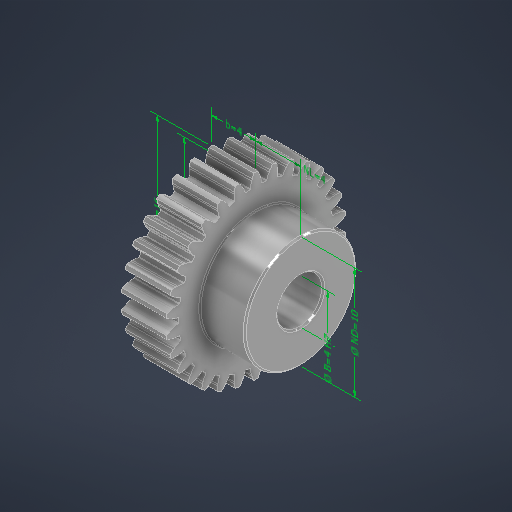
# Autodesk Inventor part: 21103000
Saved by Autodesk Inventor 2026.1 (Build 301233020, 233B)
## iProperties
Category: PARTsolutions
Company: MAEDLER
Created: 2025-12-15
Part Number: 21103000
Material: Generic
Catalog Web Link: www.3dfindit.com
Description: MAE-STZR-M0.5-MN-B4-ST-Spur Gears Made from Steel, with One-Sided Hub, Module 0.5, Tooth Width 4 mm
Vendor: MAEDLER
Document SubType Name: Modeling
Designer: psAdmin
Manufacturer: MAEDLER
Mass: 7 g
Surface Area: 9.18224 cm^2
Volume: 0.913703 cm^3
Density: 1 g/cm^3
Appearance: PSOLRGB-176-176-176
PSOL_IDENT_0: {$CADENAS_DATA/23d-libs/maedler/antriebselemente/stirnzahnraeder/stirnzahnraeder_stahl/modul_0_5_und
PSOL_IDENT_1: _0_7/stzr_m_0_5_zb4_st_mn.prj},173 {VTYP=3D},{NB=21103000},{LINA=21103000},{NN=MAE-STZR-M0.5-MN-B4-S
PSOL_IDENT_2: T},{DATE=31.10.2024 07:34:43},{GEOMDATE=31.10.2024 07:34:43},{VERSION=},{LINEID=190},{WBVAR=},{WBNUM
PSOL_IDENT_3: ERIC=}  {NB=21103000},{LINA=21103000},{KT=DUMMY},{ARTNR=21103000},{WEBSHOP=Produktdetails / Katalogs
PSOL_IDENT_4: eite / Montageanleitung},{MATK=Stahl},{MAT=Stahl 11SMn30+C (1.0715)},{M=0.5},{Z=30},{B=4},{DA=16.0},
PSOL_IDENT_5: {D=15.0},{NL=4},{ND=10},{BH7=4},{MD=5.5},{GEW=7.0},{CTN=84839089},{DIST=0.800},{GKD=14.09539},{FKD=1
PSOL_IDENT_6: 3.83300},{T0=1.57080},{UF=47.12389},{TLG=1.57080},{A=2.56515},{A3=0.85505},{PI=0.39270},{R2=0.04},{C
PSOL_IDENT_7: NSDWTEMPLATE=_dw/ansicht_right_front.dw}
NB: 21103000
NN: MAE-STZR-M0.5-MN-B4-ST
NT: Spur Gears Made from Steel, with One-Sided Hub, Module 0.5, Tooth Width 4 mm
NBSYN: $ARTNR.
LINA: 21103000
CATALOG: MÄDLER
ARTNR: 21103000
WEBSHOP: Product details / Catalogue page / Assembly instructions
MATK: Steel
MAT: Steel 11SMn30+C (1.0715)
M: 0.5
Z: 30
B: 4
DA: 16
D: 15
NL: 4
ND: 10
BH7: 4
MD: 5.5
GEW: 7
CTN: 84839089
SUPPLIER: MAEDLER
ARTICLENO: 21103000
BOMINFO: 21103000
CREATOR: CADENAS GmbH
Title: 21103000
Author: Cadenas PARTsolutions
Comments: Spur Gears Made from Steel, with One-Sided Hub, Module 0.5, Tooth Width 4 mm
Autodesk Inventor part; units mm, degrees
ref_plane "YZ Plane" through (0, 0, 0) normal (1, 0, 0) x (0, 1, 0)
ref_plane "XZ Plane" through (0, 0, 0) normal (0, 1, 0) x (-1, 0, 0)
ref_plane "XY Plane" through (0, 0, 0) normal (0, 0, 1) x (1, 0, 0)
sketch "Sketch_2" plane through (0, 0, 0) normal (0, 0, 1) x (1, 0, 0)
  line L0 (6, 0) -> (-2, 0)
  line L1 (-2, 8) -> (-2, 2.1414)
  line L2 (-2, 2.1414) -> (-1.8586, 2)
  line L3 (-1.8586, 2) -> (5.8586, 2)
  line L4 (5.8586, 2) -> (6, 2.1414)
  line L5 (6, 2.1414) -> (6, 4.8586)
  line L6 (6, 4.8586) -> (5.8586, 5)
  line L7 (5.8586, 5) -> (2.1, 5)
  arc A0 (2, 5.1) -> (2.1, 5) centre (2.1, 5.1) ccw
  line L8 (2, 5.1) -> (2, 8)
  line L9 (2, 8) -> (-2, 8)
  constraints: 20 end point, 2 point on circle, 1 centre point
revolve "Revolution1" add sketch "Sketch_2" angle 360 about axis through (6, 0, 0) along (1, 0, 0)
sketch "Sketch_4" plane through (0, 0, 0) normal (1, 0, 0) x (0, 0, -1)
  circle A0 centre (0, 0) radius 16
  arc A1 (-7.9731, -0.6556) -> (-7.9352, -1.0165) centre (0, 0) ccw
  arc A2 (-7.9352, -1.0165) -> (-7.5578, -1.1394) centre (-6.8326, 1.728) ccw
  arc A3 (-7.5578, -1.1394) -> (-7.4077, -1.1733) centre (-6.9182, 1.3448) ccw
  arc A4 (-7.4077, -1.1733) -> (-6.8456, -1.211) centre (-6.9824, 0.9573) ccw
  arc A5 (-6.8038, -1.2437) -> (-6.8456, -1.211) centre (-6.8431, -1.2509) ccw
  arc A6 (-6.8038, -1.2437) -> (-6.7214, -1.6312) centre (0, 0) ccw
  arc A7 (-6.7463, -1.6781) -> (-6.7214, -1.6312) centre (-6.7603, -1.6406) ccw
  arc A8 (-6.7463, -1.6781) -> (-7.2444, -1.9411) centre (-5.9893, -3.7146) ccw
  arc A9 (-7.2444, -1.9411) -> (-7.3678, -2.0331) centre (-5.7731, -4.0424) ccw
  arc A10 (-7.3678, -2.0331) -> (-7.6626, -2.2989) centre (-5.539, -4.3577) ccw
  arc A11 (-7.6626, -2.2989) -> (-7.5504, -2.6441) centre (0, 0) ccw
  arc A12 (-7.5504, -2.6441) -> (-7.1557, -2.6858) centre (-7.0425, 0.2697) ccw
  arc A13 (-7.1557, -2.6858) -> (-7.0019, -2.6878) centre (-7.0466, -0.123) ccw
  arc A14 (-7.0019, -2.6878) -> (-6.4443, -2.6078) centre (-7.0288, -0.5153) ccw
  arc A15 (-6.3965, -2.6311) -> (-6.4443, -2.6078) centre (-6.4335, -2.6463) ccw
  arc A16 (-6.3965, -2.6311) -> (-6.2354, -2.993) centre (0, 0) ccw
  arc A17 (-6.25, -3.0441) -> (-6.2354, -2.993) centre (-6.2715, -3.0103) ccw
  arc A18 (-6.25, -3.0441) -> (-6.6825, -3.4049) centre (-5.0861, -4.8786) ccw
  arc A19 (-6.6825, -3.4049) -> (-6.7841, -3.5206) centre (-4.8065, -5.1544) ccw
  arc A20 (-6.7841, -3.5206) -> (-7.0171, -3.8418) centre (-4.512, -5.4141) ccw
  arc A21 (-7.0171, -3.8418) -> (-6.8357, -4.1561) centre (0, 0) ccw
  arc A22 (-6.8357, -4.1561) -> (-6.4409, -4.1149) centre (-6.9447, -1.2004) ccw
  arc A23 (-6.4409, -4.1149) -> (-6.29, -4.0848) centre (-6.8671, -1.5854) ccw
  arc A24 (-6.29, -4.0848) -> (-5.7612, -3.8907) centre (-6.7681, -1.9654) ccw
  arc A25 (-5.7097, -3.9035) -> (-5.7612, -3.8907) centre (-5.7427, -3.9261) ccw
  arc A26 (-5.7097, -3.9035) -> (-5.4769, -4.224) centre (0, 0) ccw
  arc A27 (-5.4806, -4.277) -> (-5.4769, -4.224) centre (-5.5085, -4.2484) ccw
  arc A28 (-5.4806, -4.277) -> (-5.8286, -4.7199) centre (-3.9607, -5.8295) ccw
  arc A29 (-5.8286, -4.7199) -> (-5.9039, -4.8541) centre (-3.6298, -6.0411) ccw
  arc A30 (-5.9039, -4.8541) -> (-6.065, -5.2168) centre (-3.2877, -6.2339) ccw
  arc A31 (-6.065, -5.2168) -> (-5.8222, -5.4865) centre (0, 0) ccw
  arc A32 (-5.8222, -5.4865) -> (-5.4446, -5.3641) centre (-6.5434, -2.6181) ccw
  arc A33 (-5.4446, -5.3641) -> (-5.3033, -5.3033) centre (-6.3874, -2.9785) ccw
  arc A34 (-5.3033, -5.3033) -> (-4.8264, -5.0035) centre (-6.2116, -3.3296) ccw
  arc A35 (-4.7733, -5.0053) -> (-4.8264, -5.0035) centre (-4.8009, -5.0343) ccw
  arc A36 (-4.7733, -5.0053) -> (-4.479, -5.2704) centre (0, 0) ccw
  arc A37 (-4.4716, -5.323) -> (-4.479, -5.2704) centre (-4.5049, -5.3009) ccw
  arc A38 (-4.4716, -5.323) -> (-4.7199, -5.8286) centre (-2.6621, -6.5256) ccw
  arc A39 (-4.7199, -5.8286) -> (-4.7656, -5.9755) centre (-2.2945, -6.6637) ccw
  arc A40 (-4.7656, -5.9755) -> (-4.8479, -6.3638) centre (-1.9198, -6.7812) ccw
  arc A41 (-4.8479, -6.3638) -> (-4.5543, -6.5771) centre (0, 0) ccw
  arc A42 (-4.5543, -6.5771) -> (-4.2104, -6.3789) centre (-5.856, -3.9213) ccw
  arc A43 (-4.2104, -6.3789) -> (-4.0848, -6.29) centre (-5.6285, -4.2414) ccw
  arc A44 (-4.0848, -6.29) -> (-3.6807, -5.8976) centre (-5.3836, -4.5483) ccw
  arc A45 (-3.6283, -5.8884) -> (-3.6807, -5.8976) centre (-3.6493, -5.9224) ccw
  arc A46 (-3.6283, -5.8884) -> (-3.2853, -6.0864) centre (0, 0) ccw
  arc A47 (-3.2671, -6.1364) -> (-3.2853, -6.0864) centre (-3.3043, -6.1216) ccw
  arc A48 (-3.2671, -6.1364) -> (-3.4049, -6.6825) centre (-1.2472, -6.9365) ccw
  arc A49 (-3.4049, -6.6825) -> (-3.4191, -6.8358) centre (-0.8589, -6.9952) ccw
  arc A50 (-3.4191, -6.8358) -> (-3.4188, -7.2327) centre (-0.4679, -7.0321) ccw
  arc A51 (-3.4188, -7.2327) -> (-3.0873, -7.3803) centre (0, 0) ccw
  arc A52 (-3.0873, -7.3803) -> (-2.7921, -7.1149) centre (-4.9128, -5.0532) ccw
  arc A53 (-2.7921, -7.1149) -> (-2.6878, -7.0019) centre (-4.6237, -5.319) ccw
  arc A54 (-2.6878, -7.0019) -> (-2.3741, -6.534) centre (-4.3203, -5.5682) ccw
  arc A55 (-2.3248, -6.5141) -> (-2.3741, -6.534) centre (-2.3382, -6.5518) ccw
  arc A56 (-2.3248, -6.5141) -> (-1.9481, -6.6365) centre (0, 0) ccw
  arc A57 (-1.9199, -6.6815) -> (-1.9481, -6.6365) centre (-1.9594, -6.6749) ccw
  arc A58 (-1.9199, -6.6815) -> (-1.9411, -7.2444) centre (0.2222, -7.0442) ccw
  arc A59 (-1.9411, -7.2444) -> (-1.9231, -7.3973) centre (0.6142, -7.0209) ccw
  arc A60 (-1.9231, -7.3973) -> (-1.8403, -7.7854) centre (1.0043, -6.9758) ccw
  arc A61 (-1.8403, -7.7854) -> (-1.4854, -7.8609) centre (0, 0) ccw
  arc A62 (-1.4854, -7.8609) -> (-1.2519, -7.5399) centre (-3.7548, -5.9642) ccw
  arc A63 (-1.2519, -7.5399) -> (-1.1733, -7.4077) centre (-3.4168, -6.1641) ccw
  arc A64 (-1.1733, -7.4077) -> (-0.9637, -6.8848) centre (-3.0682, -6.3448) ccw
  arc A65 (-0.9196, -6.8551) -> (-0.9637, -6.8848) centre (-0.925, -6.8947) ccw
  arc A66 (-0.9196, -6.8551) -> (-0.5257, -6.8965) centre (0, 0) ccw
  arc A67 (-0.4888, -6.9347) -> (-0.5257, -6.8965) centre (-0.5288, -6.9364) ccw
  arc A68 (-0.4888, -6.9347) -> (-0.3925, -7.4897) centre (1.682, -6.8441) ccw
  arc A69 (-0.3925, -7.4897) -> (-0.3431, -7.6355) centre (2.0605, -6.7397) ccw
  arc A70 (-0.3431, -7.6355) -> (-0.1814, -7.9979) centre (2.4327, -6.6145) ccw
  arc A71 (-0.1814, -7.9979) -> (0.1814, -7.9979) centre (0, 0) ccw
  arc A72 (0.1814, -7.9979) -> (0.3431, -7.6355) centre (-2.4327, -6.6145) ccw
  arc A73 (0.3431, -7.6355) -> (0.3925, -7.4897) centre (-2.0605, -6.7397) ccw
  arc A74 (0.3925, -7.4897) -> (0.4888, -6.9347) centre (-1.682, -6.8441) ccw
  arc A75 (0.5257, -6.8965) -> (0.4888, -6.9347) centre (0.5288, -6.9364) ccw
  arc A76 (0.5257, -6.8965) -> (0.9196, -6.8551) centre (0, 0) ccw
  arc A77 (0.9637, -6.8848) -> (0.9196, -6.8551) centre (0.925, -6.8947) ccw
  arc A78 (0.9637, -6.8848) -> (1.1733, -7.4077) centre (3.0682, -6.3448) ccw
  arc A79 (1.1733, -7.4077) -> (1.2519, -7.5399) centre (3.4168, -6.1641) ccw
  arc A80 (1.2519, -7.5399) -> (1.4854, -7.8609) centre (3.7548, -5.9642) ccw
  arc A81 (1.4854, -7.8609) -> (1.8403, -7.7854) centre (0, 0) ccw
  arc A82 (1.8403, -7.7854) -> (1.9231, -7.3973) centre (-1.0043, -6.9758) ccw
  arc A83 (1.9231, -7.3973) -> (1.9411, -7.2444) centre (-0.6142, -7.0209) ccw
  arc A84 (1.9411, -7.2444) -> (1.9199, -6.6815) centre (-0.2222, -7.0442) ccw
  arc A85 (1.9481, -6.6365) -> (1.9199, -6.6815) centre (1.9594, -6.6749) ccw
  arc A86 (1.9481, -6.6365) -> (2.3248, -6.5141) centre (0, 0) ccw
  arc A87 (2.3741, -6.534) -> (2.3248, -6.5141) centre (2.3382, -6.5518) ccw
  arc A88 (2.3741, -6.534) -> (2.6878, -7.0019) centre (4.3203, -5.5682) ccw
  arc A89 (2.6878, -7.0019) -> (2.7921, -7.1149) centre (4.6237, -5.319) ccw
  arc A90 (2.7921, -7.1149) -> (3.0873, -7.3803) centre (4.9128, -5.0532) ccw
  arc A91 (3.0873, -7.3803) -> (3.4188, -7.2327) centre (0, 0) ccw
  arc A92 (3.4188, -7.2327) -> (3.4191, -6.8358) centre (0.4679, -7.0321) ccw
  arc A93 (3.4191, -6.8358) -> (3.4049, -6.6825) centre (0.8589, -6.9952) ccw
  arc A94 (3.4049, -6.6825) -> (3.2671, -6.1364) centre (1.2472, -6.9365) ccw
  arc A95 (3.2853, -6.0864) -> (3.2671, -6.1364) centre (3.3043, -6.1216) ccw
  arc A96 (3.2853, -6.0864) -> (3.6283, -5.8884) centre (0, 0) ccw
  arc A97 (3.6807, -5.8976) -> (3.6283, -5.8884) centre (3.6493, -5.9224) ccw
  arc A98 (3.6807, -5.8976) -> (4.0848, -6.29) centre (5.3836, -4.5483) ccw
  arc A99 (4.0848, -6.29) -> (4.2104, -6.3789) centre (5.6285, -4.2414) ccw
  arc A100 (4.2104, -6.3789) -> (4.5543, -6.5771) centre (5.856, -3.9213) ccw
  arc A101 (4.5543, -6.5771) -> (4.8479, -6.3638) centre (0, 0) ccw
  arc A102 (4.8479, -6.3638) -> (4.7656, -5.9755) centre (1.9198, -6.7812) ccw
  arc A103 (4.7656, -5.9755) -> (4.7199, -5.8286) centre (2.2945, -6.6637) ccw
  arc A104 (4.7199, -5.8286) -> (4.4716, -5.323) centre (2.6621, -6.5256) ccw
  arc A105 (4.479, -5.2704) -> (4.4716, -5.323) centre (4.5049, -5.3009) ccw
  arc A106 (4.479, -5.2704) -> (4.7733, -5.0053) centre (0, 0) ccw
  arc A107 (4.8264, -5.0035) -> (4.7733, -5.0053) centre (4.8009, -5.0343) ccw
  arc A108 (4.8264, -5.0035) -> (5.3033, -5.3033) centre (6.2116, -3.3296) ccw
  arc A109 (5.3033, -5.3033) -> (5.4446, -5.3641) centre (6.3874, -2.9785) ccw
  arc A110 (5.4446, -5.3641) -> (5.8222, -5.4865) centre (6.5434, -2.6181) ccw
  arc A111 (5.8222, -5.4865) -> (6.065, -5.2168) centre (0, 0) ccw
  arc A112 (6.065, -5.2168) -> (5.9039, -4.8541) centre (3.2877, -6.2339) ccw
  arc A113 (5.9039, -4.8541) -> (5.8286, -4.7199) centre (3.6298, -6.0411) ccw
  arc A114 (5.8286, -4.7199) -> (5.4806, -4.277) centre (3.9607, -5.8295) ccw
  arc A115 (5.4769, -4.224) -> (5.4806, -4.277) centre (5.5085, -4.2484) ccw
  arc A116 (5.4769, -4.224) -> (5.7097, -3.9035) centre (0, 0) ccw
  arc A117 (5.7612, -3.8907) -> (5.7097, -3.9035) centre (5.7427, -3.9261) ccw
  arc A118 (5.7612, -3.8907) -> (6.29, -4.0848) centre (6.7681, -1.9654) ccw
  arc A119 (6.29, -4.0848) -> (6.4409, -4.1149) centre (6.8671, -1.5854) ccw
  arc A120 (6.4409, -4.1149) -> (6.8357, -4.1561) centre (6.9447, -1.2004) ccw
  arc A121 (6.8357, -4.1561) -> (7.0171, -3.8418) centre (0, 0) ccw
  arc A122 (7.0171, -3.8418) -> (6.7841, -3.5206) centre (4.512, -5.4141) ccw
  arc A123 (6.7841, -3.5206) -> (6.6825, -3.4049) centre (4.8065, -5.1544) ccw
  arc A124 (6.6825, -3.4049) -> (6.25, -3.0441) centre (5.0861, -4.8786) ccw
  arc A125 (6.2354, -2.993) -> (6.25, -3.0441) centre (6.2715, -3.0103) ccw
  arc A126 (6.2354, -2.993) -> (6.3965, -2.6311) centre (0, 0) ccw
  arc A127 (6.4443, -2.6078) -> (6.3965, -2.6311) centre (6.4335, -2.6463) ccw
  arc A128 (6.4443, -2.6078) -> (7.0019, -2.6878) centre (7.0288, -0.5153) ccw
  arc A129 (7.0019, -2.6878) -> (7.1557, -2.6858) centre (7.0466, -0.123) ccw
  arc A130 (7.1557, -2.6858) -> (7.5504, -2.6441) centre (7.0425, 0.2697) ccw
  arc A131 (7.5504, -2.6441) -> (7.6626, -2.2989) centre (0, 0) ccw
  arc A132 (7.6626, -2.2989) -> (7.3678, -2.0331) centre (5.539, -4.3577) ccw
  arc A133 (7.3678, -2.0331) -> (7.2444, -1.9411) centre (5.7731, -4.0424) ccw
  arc A134 (7.2444, -1.9411) -> (6.7463, -1.6781) centre (5.9893, -3.7146) ccw
  arc A135 (6.7214, -1.6312) -> (6.7463, -1.6781) centre (6.7603, -1.6406) ccw
  arc A136 (6.7214, -1.6312) -> (6.8038, -1.2437) centre (0, 0) ccw
  arc A137 (6.8456, -1.211) -> (6.8038, -1.2437) centre (6.8431, -1.2509) ccw
  arc A138 (6.8456, -1.211) -> (7.4077, -1.1733) centre (6.9824, 0.9573) ccw
  arc A139 (7.4077, -1.1733) -> (7.5578, -1.1394) centre (6.9182, 1.3448) ccw
  arc A140 (7.5578, -1.1394) -> (7.9352, -1.0165) centre (6.8326, 1.728) ccw
  arc A141 (7.9352, -1.0165) -> (7.9731, -0.6556) centre (0, 0) ccw
  arc A142 (7.9731, -0.6556) -> (7.6295, -0.4569) centre (6.324, -3.1108) ccw
  arc A143 (7.6295, -0.4569) -> (7.4897, -0.3925) centre (6.4874, -2.7538) ccw
  arc A144 (7.4897, -0.3925) -> (6.9478, -0.2388) centre (6.6307, -2.3881) ccw
  arc A145 (6.9137, -0.198) -> (6.9478, -0.2388) centre (6.9536, -0.1992) ccw
  arc A146 (6.9137, -0.198) -> (6.9137, 0.198) centre (0, 0) ccw
  arc A147 (6.9478, 0.2388) -> (6.9137, 0.198) centre (6.9536, 0.1992) ccw
  arc A148 (6.9478, 0.2388) -> (7.4897, 0.3925) centre (6.6307, 2.3881) ccw
  arc A149 (7.4897, 0.3925) -> (7.6295, 0.4569) centre (6.4874, 2.7538) ccw
  arc A150 (7.6295, 0.4569) -> (7.9731, 0.6556) centre (6.324, 3.1108) ccw
  arc A151 (7.9731, 0.6556) -> (7.9352, 1.0165) centre (0, 0) ccw
  arc A152 (7.9352, 1.0165) -> (7.5578, 1.1394) centre (6.8326, -1.728) ccw
  arc A153 (7.5578, 1.1394) -> (7.4077, 1.1733) centre (6.9182, -1.3448) ccw
  arc A154 (7.4077, 1.1733) -> (6.8456, 1.211) centre (6.9824, -0.9573) ccw
  arc A155 (6.8038, 1.2437) -> (6.8456, 1.211) centre (6.8431, 1.2509) ccw
  arc A156 (6.8038, 1.2437) -> (6.7214, 1.6312) centre (0, 0) ccw
  arc A157 (6.7463, 1.6781) -> (6.7214, 1.6312) centre (6.7603, 1.6406) ccw
  arc A158 (6.7463, 1.6781) -> (7.2444, 1.9411) centre (5.9893, 3.7146) ccw
  arc A159 (7.2444, 1.9411) -> (7.3678, 2.0331) centre (5.7731, 4.0424) ccw
  arc A160 (7.3678, 2.0331) -> (7.6626, 2.2989) centre (5.539, 4.3577) ccw
  arc A161 (7.6626, 2.2989) -> (7.5504, 2.6441) centre (0, 0) ccw
  arc A162 (7.5504, 2.6441) -> (7.1557, 2.6858) centre (7.0425, -0.2697) ccw
  arc A163 (7.1557, 2.6858) -> (7.0019, 2.6878) centre (7.0466, 0.123) ccw
  arc A164 (7.0019, 2.6878) -> (6.4443, 2.6078) centre (7.0288, 0.5153) ccw
  arc A165 (6.3965, 2.6311) -> (6.4443, 2.6078) centre (6.4335, 2.6463) ccw
  arc A166 (6.3965, 2.6311) -> (6.2354, 2.993) centre (0, 0) ccw
  arc A167 (6.25, 3.0441) -> (6.2354, 2.993) centre (6.2715, 3.0103) ccw
  arc A168 (6.25, 3.0441) -> (6.6825, 3.4049) centre (5.0861, 4.8786) ccw
  arc A169 (6.6825, 3.4049) -> (6.7841, 3.5206) centre (4.8065, 5.1544) ccw
  arc A170 (6.7841, 3.5206) -> (7.0171, 3.8418) centre (4.512, 5.4141) ccw
  arc A171 (7.0171, 3.8418) -> (6.8357, 4.1561) centre (0, 0) ccw
  arc A172 (6.8357, 4.1561) -> (6.4409, 4.1149) centre (6.9447, 1.2004) ccw
  arc A173 (6.4409, 4.1149) -> (6.29, 4.0848) centre (6.8671, 1.5854) ccw
  arc A174 (6.29, 4.0848) -> (5.7612, 3.8907) centre (6.7681, 1.9654) ccw
  arc A175 (5.7097, 3.9035) -> (5.7612, 3.8907) centre (5.7427, 3.9261) ccw
  arc A176 (5.7097, 3.9035) -> (5.4769, 4.224) centre (0, 0) ccw
  arc A177 (5.4806, 4.277) -> (5.4769, 4.224) centre (5.5085, 4.2484) ccw
  arc A178 (5.4806, 4.277) -> (5.8286, 4.7199) centre (3.9607, 5.8295) ccw
  arc A179 (5.8286, 4.7199) -> (5.9039, 4.8541) centre (3.6298, 6.0411) ccw
  arc A180 (5.9039, 4.8541) -> (6.065, 5.2168) centre (3.2877, 6.2339) ccw
  arc A181 (6.065, 5.2168) -> (5.8222, 5.4865) centre (0, 0) ccw
  arc A182 (5.8222, 5.4865) -> (5.4446, 5.3641) centre (6.5434, 2.6181) ccw
  arc A183 (5.4446, 5.3641) -> (5.3033, 5.3033) centre (6.3874, 2.9785) ccw
  arc A184 (5.3033, 5.3033) -> (4.8264, 5.0035) centre (6.2116, 3.3296) ccw
  arc A185 (4.7733, 5.0053) -> (4.8264, 5.0035) centre (4.8009, 5.0343) ccw
  arc A186 (4.7733, 5.0053) -> (4.479, 5.2704) centre (0, 0) ccw
  arc A187 (4.4716, 5.323) -> (4.479, 5.2704) centre (4.5049, 5.3009) ccw
  arc A188 (4.4716, 5.323) -> (4.7199, 5.8286) centre (2.6621, 6.5256) ccw
  arc A189 (4.7199, 5.8286) -> (4.7656, 5.9755) centre (2.2945, 6.6637) ccw
  arc A190 (4.7656, 5.9755) -> (4.8479, 6.3638) centre (1.9198, 6.7812) ccw
  arc A191 (4.8479, 6.3638) -> (4.5543, 6.5771) centre (0, 0) ccw
  arc A192 (4.5543, 6.5771) -> (4.2104, 6.3789) centre (5.856, 3.9213) ccw
  arc A193 (4.2104, 6.3789) -> (4.0848, 6.29) centre (5.6285, 4.2414) ccw
  arc A194 (4.0848, 6.29) -> (3.6807, 5.8976) centre (5.3836, 4.5483) ccw
  arc A195 (3.6283, 5.8884) -> (3.6807, 5.8976) centre (3.6493, 5.9224) ccw
  arc A196 (3.6283, 5.8884) -> (3.2853, 6.0864) centre (0, 0) ccw
  arc A197 (3.2671, 6.1364) -> (3.2853, 6.0864) centre (3.3043, 6.1216) ccw
  arc A198 (3.2671, 6.1364) -> (3.4049, 6.6825) centre (1.2472, 6.9365) ccw
  arc A199 (3.4049, 6.6825) -> (3.4191, 6.8358) centre (0.8589, 6.9952) ccw
  arc A200 (3.4191, 6.8358) -> (3.4188, 7.2327) centre (0.4679, 7.0321) ccw
  arc A201 (3.4188, 7.2327) -> (3.0873, 7.3803) centre (0, 0) ccw
  arc A202 (3.0873, 7.3803) -> (2.7921, 7.1149) centre (4.9128, 5.0532) ccw
  arc A203 (2.7921, 7.1149) -> (2.6878, 7.0019) centre (4.6237, 5.319) ccw
  arc A204 (2.6878, 7.0019) -> (2.3741, 6.534) centre (4.3203, 5.5682) ccw
  arc A205 (2.3248, 6.5141) -> (2.3741, 6.534) centre (2.3382, 6.5518) ccw
  arc A206 (2.3248, 6.5141) -> (1.9481, 6.6365) centre (0, 0) ccw
  arc A207 (1.9199, 6.6815) -> (1.9481, 6.6365) centre (1.9594, 6.6749) ccw
  arc A208 (1.9199, 6.6815) -> (1.9411, 7.2444) centre (-0.2222, 7.0442) ccw
  arc A209 (1.9411, 7.2444) -> (1.9231, 7.3973) centre (-0.6142, 7.0209) ccw
  arc A210 (1.9231, 7.3973) -> (1.8403, 7.7854) centre (-1.0043, 6.9758) ccw
  arc A211 (1.8403, 7.7854) -> (1.4854, 7.8609) centre (0, 0) ccw
  arc A212 (1.4854, 7.8609) -> (1.2519, 7.5399) centre (3.7548, 5.9642) ccw
  arc A213 (1.2519, 7.5399) -> (1.1733, 7.4077) centre (3.4168, 6.1641) ccw
  arc A214 (1.1733, 7.4077) -> (0.9637, 6.8848) centre (3.0682, 6.3448) ccw
  arc A215 (0.9196, 6.8551) -> (0.9637, 6.8848) centre (0.925, 6.8947) ccw
  arc A216 (0.9196, 6.8551) -> (0.5257, 6.8965) centre (0, 0) ccw
  arc A217 (0.4888, 6.9347) -> (0.5257, 6.8965) centre (0.5288, 6.9364) ccw
  arc A218 (0.4888, 6.9347) -> (0.3925, 7.4897) centre (-1.682, 6.8441) ccw
  arc A219 (0.3925, 7.4897) -> (0.3431, 7.6355) centre (-2.0605, 6.7397) ccw
  arc A220 (0.3431, 7.6355) -> (0.1814, 7.9979) centre (-2.4327, 6.6145) ccw
  arc A221 (0.1814, 7.9979) -> (-0.1814, 7.9979) centre (0, 0) ccw
  arc A222 (-0.1814, 7.9979) -> (-0.3431, 7.6355) centre (2.4327, 6.6145) ccw
  arc A223 (-0.3431, 7.6355) -> (-0.3925, 7.4897) centre (2.0605, 6.7397) ccw
  arc A224 (-0.3925, 7.4897) -> (-0.4888, 6.9347) centre (1.682, 6.8441) ccw
  arc A225 (-0.5257, 6.8965) -> (-0.4888, 6.9347) centre (-0.5288, 6.9364) ccw
  arc A226 (-0.5257, 6.8965) -> (-0.9196, 6.8551) centre (0, 0) ccw
  arc A227 (-0.9637, 6.8848) -> (-0.9196, 6.8551) centre (-0.925, 6.8947) ccw
  arc A228 (-0.9637, 6.8848) -> (-1.1733, 7.4077) centre (-3.0682, 6.3448) ccw
  arc A229 (-1.1733, 7.4077) -> (-1.2519, 7.5399) centre (-3.4168, 6.1641) ccw
  arc A230 (-1.2519, 7.5399) -> (-1.4854, 7.8609) centre (-3.7548, 5.9642) ccw
  arc A231 (-1.4854, 7.8609) -> (-1.8403, 7.7854) centre (0, 0) ccw
  arc A232 (-1.8403, 7.7854) -> (-1.9231, 7.3973) centre (1.0043, 6.9758) ccw
  arc A233 (-1.9231, 7.3973) -> (-1.9411, 7.2444) centre (0.6142, 7.0209) ccw
  arc A234 (-1.9411, 7.2444) -> (-1.9199, 6.6815) centre (0.2222, 7.0442) ccw
  arc A235 (-1.9481, 6.6365) -> (-1.9199, 6.6815) centre (-1.9594, 6.6749) ccw
  arc A236 (-1.9481, 6.6365) -> (-2.3248, 6.5141) centre (0, 0) ccw
  arc A237 (-2.3741, 6.534) -> (-2.3248, 6.5141) centre (-2.3382, 6.5518) ccw
  arc A238 (-2.3741, 6.534) -> (-2.6878, 7.0019) centre (-4.3203, 5.5682) ccw
  arc A239 (-2.6878, 7.0019) -> (-2.7921, 7.1149) centre (-4.6237, 5.319) ccw
  arc A240 (-2.7921, 7.1149) -> (-3.0873, 7.3803) centre (-4.9128, 5.0532) ccw
  arc A241 (-3.0873, 7.3803) -> (-3.4188, 7.2327) centre (0, 0) ccw
  arc A242 (-3.4188, 7.2327) -> (-3.4191, 6.8358) centre (-0.4679, 7.0321) ccw
  arc A243 (-3.4191, 6.8358) -> (-3.4049, 6.6825) centre (-0.8589, 6.9952) ccw
  arc A244 (-3.4049, 6.6825) -> (-3.2671, 6.1364) centre (-1.2472, 6.9365) ccw
  arc A245 (-3.2853, 6.0864) -> (-3.2671, 6.1364) centre (-3.3043, 6.1216) ccw
  arc A246 (-3.2853, 6.0864) -> (-3.6283, 5.8884) centre (0, 0) ccw
  arc A247 (-3.6807, 5.8976) -> (-3.6283, 5.8884) centre (-3.6493, 5.9224) ccw
  arc A248 (-3.6807, 5.8976) -> (-4.0848, 6.29) centre (-5.3836, 4.5483) ccw
  arc A249 (-4.0848, 6.29) -> (-4.2104, 6.3789) centre (-5.6285, 4.2414) ccw
  arc A250 (-4.2104, 6.3789) -> (-4.5543, 6.5771) centre (-5.856, 3.9213) ccw
  arc A251 (-4.5543, 6.5771) -> (-4.8479, 6.3638) centre (0, 0) ccw
  arc A252 (-4.8479, 6.3638) -> (-4.7656, 5.9755) centre (-1.9198, 6.7812) ccw
  arc A253 (-4.7656, 5.9755) -> (-4.7199, 5.8286) centre (-2.2945, 6.6637) ccw
  arc A254 (-4.7199, 5.8286) -> (-4.4716, 5.323) centre (-2.6621, 6.5256) ccw
  arc A255 (-4.479, 5.2704) -> (-4.4716, 5.323) centre (-4.5049, 5.3009) ccw
  arc A256 (-4.479, 5.2704) -> (-4.7733, 5.0053) centre (0, 0) ccw
  arc A257 (-4.8264, 5.0035) -> (-4.7733, 5.0053) centre (-4.8009, 5.0343) ccw
  arc A258 (-4.8264, 5.0035) -> (-5.3033, 5.3033) centre (-6.2116, 3.3296) ccw
  arc A259 (-5.3033, 5.3033) -> (-5.4446, 5.3641) centre (-6.3874, 2.9785) ccw
  arc A260 (-5.4446, 5.3641) -> (-5.8222, 5.4865) centre (-6.5434, 2.6181) ccw
  arc A261 (-5.8222, 5.4865) -> (-6.065, 5.2168) centre (0, 0) ccw
  arc A262 (-6.065, 5.2168) -> (-5.9039, 4.8541) centre (-3.2877, 6.2339) ccw
  arc A263 (-5.9039, 4.8541) -> (-5.8286, 4.7199) centre (-3.6298, 6.0411) ccw
  arc A264 (-5.8286, 4.7199) -> (-5.4806, 4.277) centre (-3.9607, 5.8295) ccw
  arc A265 (-5.4769, 4.224) -> (-5.4806, 4.277) centre (-5.5085, 4.2484) ccw
  arc A266 (-5.4769, 4.224) -> (-5.7097, 3.9035) centre (0, 0) ccw
  arc A267 (-5.7612, 3.8907) -> (-5.7097, 3.9035) centre (-5.7427, 3.9261) ccw
  arc A268 (-5.7612, 3.8907) -> (-6.29, 4.0848) centre (-6.7681, 1.9654) ccw
  arc A269 (-6.29, 4.0848) -> (-6.4409, 4.1149) centre (-6.8671, 1.5854) ccw
  arc A270 (-6.4409, 4.1149) -> (-6.8357, 4.1561) centre (-6.9447, 1.2004) ccw
  arc A271 (-6.8357, 4.1561) -> (-7.0171, 3.8418) centre (0, 0) ccw
  arc A272 (-7.0171, 3.8418) -> (-6.7841, 3.5206) centre (-4.512, 5.4141) ccw
  arc A273 (-6.7841, 3.5206) -> (-6.6825, 3.4049) centre (-4.8065, 5.1544) ccw
  arc A274 (-6.6825, 3.4049) -> (-6.25, 3.0441) centre (-5.0861, 4.8786) ccw
  arc A275 (-6.2354, 2.993) -> (-6.25, 3.0441) centre (-6.2715, 3.0103) ccw
  arc A276 (-6.2354, 2.993) -> (-6.3965, 2.6311) centre (0, 0) ccw
  arc A277 (-6.4443, 2.6078) -> (-6.3965, 2.6311) centre (-6.4335, 2.6463) ccw
  arc A278 (-6.4443, 2.6078) -> (-7.0019, 2.6878) centre (-7.0288, 0.5153) ccw
  arc A279 (-7.0019, 2.6878) -> (-7.1557, 2.6858) centre (-7.0466, 0.123) ccw
  arc A280 (-7.1557, 2.6858) -> (-7.5504, 2.6441) centre (-7.0425, -0.2697) ccw
  arc A281 (-7.5504, 2.6441) -> (-7.6626, 2.2989) centre (0, 0) ccw
  arc A282 (-7.6626, 2.2989) -> (-7.3678, 2.0331) centre (-5.539, 4.3577) ccw
  arc A283 (-7.3678, 2.0331) -> (-7.2444, 1.9411) centre (-5.7731, 4.0424) ccw
  arc A284 (-7.2444, 1.9411) -> (-6.7463, 1.6781) centre (-5.9893, 3.7146) ccw
  arc A285 (-6.7214, 1.6312) -> (-6.7463, 1.6781) centre (-6.7603, 1.6406) ccw
  arc A286 (-6.7214, 1.6312) -> (-6.8038, 1.2437) centre (0, 0) ccw
  arc A287 (-6.8456, 1.211) -> (-6.8038, 1.2437) centre (-6.8431, 1.2509) ccw
  arc A288 (-6.8456, 1.211) -> (-7.4077, 1.1733) centre (-6.9824, -0.9573) ccw
  arc A289 (-7.4077, 1.1733) -> (-7.5578, 1.1394) centre (-6.9182, -1.3448) ccw
  arc A290 (-7.5578, 1.1394) -> (-7.9352, 1.0165) centre (-6.8326, -1.728) ccw
  arc A291 (-7.9352, 1.0165) -> (-7.9731, 0.6556) centre (0, 0) ccw
  arc A292 (-7.9731, 0.6556) -> (-7.6295, 0.4569) centre (-6.324, 3.1108) ccw
  arc A293 (-7.6295, 0.4569) -> (-7.4897, 0.3925) centre (-6.4874, 2.7538) ccw
  arc A294 (-7.4897, 0.3925) -> (-6.9478, 0.2388) centre (-6.6307, 2.3881) ccw
  arc A295 (-6.9137, 0.198) -> (-6.9478, 0.2388) centre (-6.9536, 0.1992) ccw
  arc A296 (-6.9137, 0.198) -> (-6.9137, -0.198) centre (0, 0) ccw
  arc A297 (-6.9478, -0.2388) -> (-6.9137, -0.198) centre (-6.9536, -0.1992) ccw
  arc A298 (-6.9478, -0.2388) -> (-7.4897, -0.3925) centre (-6.6307, -2.3881) ccw
  arc A299 (-7.4897, -0.3925) -> (-7.6295, -0.4569) centre (-6.4874, -2.7538) ccw
  arc A300 (-7.6295, -0.4569) -> (-7.9731, -0.6556) centre (-6.324, -3.1108) ccw
  constraints: 600 point on circle, 301 centre point
extrude "Extrusion1" cut sketch "Sketch_4" along normal mid plane 4
body "Solid1"
